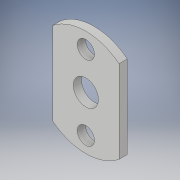
# Autodesk Inventor part: Part12
Saved by Autodesk Inventor 2019 (Build 230136000, 136)
## iProperties
Created: 2018-09-18
Part Number: Part12
Material: Generic
Document SubType Name: Modeling
Designer: drawing
Density: 1 g/cm^3
Appearance: Default
Author: drawing
Autodesk Inventor part; units mm, degrees
ref_plane "YZ Plane" through (0, 0, 0) normal (1, 0, 0) x (0, 1, 0)
ref_plane "XZ Plane" through (0, 0, 0) normal (0, 1, 0) x (-1, 0, 0)
ref_plane "XY Plane" through (0, 0, 0) normal (0, 0, 1) x (1, 0, 0)
sketch "Sketch1" plane through (0, 0, 0) normal (0, 0, 1) x (1, 0, 0)
  circle A0 centre (0, 0) radius 20.32
  dimension "d0" = 40.64
  constraints: 1 centre point, 1 coincident
  measures "d0" diameter of A0
extrude "Extrusion1" add sketch "Sketch1" along normal blind 3.175
sketch "Sketch2" plane through (0, 0, 3.175) normal (0, 0, 1) x (1, 0, 0)
  point P0 (0, 0)
  point P1 (0, 0)
  constraints: 1 coincident
hole "Hole1" at (0, 0, 3.175) direction (0, 0, -1) diameter 9.652 depth 10.9728 tip angle 118
sketch "Sketch3" plane through (0, 0, 3.175) normal (0, 0, 1) x (1, 0, 0)
  point P0 (0, 0)
  point P1 (0, 14.2875)
  point P2 (0, -14.2875)
  dimension "d10" = 28.575
  dimension "d11" = 14.2875
  constraints: 2 vertical alignment
  measures "d10" distance of point (0, 14.287) point (0, -14.287)
  measures "d11" distance of point (0, 0) point (0, 14.287)
hole "Hole2" at (0, 14.2875, 3.175) at (0, -14.2875, 3.175) direction (0, 0, -1) diameter 6.604 depth 10.9728 tip angle 118
sketch "Sketch4" plane through (0, 0, 3.175) normal (0, 0, 1) x (1, 0, 0)
  line L0 (-12.7, -38.2443) -> (12.7, -38.2443)
  line L1 (12.7, -38.2443) -> (12.7, 37.8114)
  line L2 (12.7, 37.8114) -> (-12.7, 37.8114)
  line L3 (-12.7, 37.8114) -> (-12.7, -38.2443)
  line L4 (-54.4025, 52.7865) -> (43.8573, 52.7865)
  line L5 (43.8573, 52.7865) -> (43.8573, -66.4941)
  line L6 (43.8573, -66.4941) -> (-54.4025, -66.4941)
  line L7 (-54.4025, -66.4941) -> (-54.4025, 52.7865)
  point P0 (0, 0)
  dimension "d19" = 25.4
  dimension "d20" = 12.7
  constraints: 16 end point, 4 parallel, 2 horizontal, 2 perpendicular
  measures "d19" distance of L1.end L2.end
  measures "d20" distance from line of L3 point (0, 0)
extrude "Extrusion2" cut sketch "Sketch4" against normal blind 3.175
equation "\"d11\" = 0.5 * d10"
equation "\"d20\" = 0.5 * d19"
body "Solid1"
